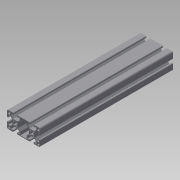
# Autodesk Inventor part: 1530-ULS
Saved by Autodesk Inventor 2013 (Build 170138000, 138)
## iProperties
Created: 2014-04-23
Part Number: 1530-ULS
Material: Generic
Document SubType Name: Modeling
Density: 1 g/cm^3
Vendor: 80/20 Inc.
Engineer: Ross Bowman
Designer: Ross Bowman
Catalog Web Link: 8020.net
Company: 80/20 Inc.
Author: Ross Bowman
Keywords: 80/20 , 8020 , T-Slot , Extrusion
Material: 6105-T5 Aluminum
Autodesk Inventor part; units mm, degrees
ref_plane "YZ Plane" through (0, 0, 0) normal (1, 0, 0) x (0, 1, 0)
ref_plane "XZ Plane" through (0, 0, 0) normal (0, 1, 0) x (-1, 0, 0)
ref_plane "XY Plane" through (0, 0, 0) normal (0, 0, 1) x (1, 0, 0)
sketch "Sketch1" plane through (0, 0, 0) normal (0, 0, 1) x (1, 0, 0)
  arc A0 (30.9118, 12.2428) -> (31.2928, 11.8618) centre (31.2928, 12.2428) ccw
  line L0 (30.9118, 16.8656) -> (30.9118, 12.2428)
  arc A1 (31.2928, 17.2466) -> (30.9118, 16.8656) centre (31.2928, 16.8656) ccw
  line L1 (33.5026, 17.2466) -> (31.2928, 17.2466)
  arc A2 (36.2966, 14.4526) -> (33.5026, 17.2466) centre (33.5026, 14.4526) ccw
  line L2 (36.2966, 12.2428) -> (36.2966, 14.4526)
  arc A3 (35.9156, 11.8618) -> (36.2966, 12.2428) centre (35.9156, 12.2428) ccw
  line L3 (31.2928, 11.8618) -> (35.9156, 11.8618)
  arc A4 (22.1619, -1.178) -> (22.1619, 1.178) centre (19.05, 0) ccw
  arc A5 (22.1619, -1.178) -> (22.2488, -1.5823) centre (22.5182, -1.3129) ccw
  line L4 (23.9585, -3.2921) -> (22.2488, -1.5823)
  arc A6 (24.2189, -3.9207) -> (23.9585, -3.2921) centre (23.3299, -3.9207) ccw
  line L5 (24.2189, -4.9149) -> (24.2189, -3.9207)
  arc A7 (23.9649, -5.1689) -> (24.2189, -4.9149) centre (23.9649, -4.9149) ccw
  line L6 (22.9707, -5.1689) -> (23.9649, -5.1689)
  arc A8 (22.3421, -4.9085) -> (22.9707, -5.1689) centre (22.9707, -4.2799) ccw
  line L7 (20.6323, -3.1988) -> (22.3421, -4.9085)
  arc A9 (20.6323, -3.1988) -> (20.228, -3.1119) centre (20.3629, -3.4682) ccw
  arc A10 (17.872, -3.1119) -> (20.228, -3.1119) centre (19.05, 0) ccw
  arc A11 (17.872, -3.1119) -> (17.4677, -3.1988) centre (17.7371, -3.4682) ccw
  line L8 (15.7579, -4.9085) -> (17.4677, -3.1988)
  arc A12 (15.1293, -5.1689) -> (15.7579, -4.9085) centre (15.1293, -4.2799) ccw
  line L9 (14.1351, -5.1689) -> (15.1293, -5.1689)
  arc A13 (13.8811, -4.9149) -> (14.1351, -5.1689) centre (14.1351, -4.9149) ccw
  line L10 (13.8811, -3.9207) -> (13.8811, -4.9149)
  arc A14 (14.1415, -3.2921) -> (13.8811, -3.9207) centre (14.7701, -3.9207) ccw
  line L11 (15.8512, -1.5823) -> (14.1415, -3.2921)
  arc A15 (15.8512, -1.5823) -> (15.9381, -1.178) centre (15.5818, -1.3129) ccw
  arc A16 (15.9381, 1.178) -> (15.9381, -1.178) centre (19.05, 0) ccw
  arc A17 (15.9381, 1.178) -> (15.8512, 1.5823) centre (15.5818, 1.3129) ccw
  line L12 (14.1415, 3.2921) -> (15.8512, 1.5823)
  arc A18 (13.8811, 3.9207) -> (14.1415, 3.2921) centre (14.7701, 3.9207) ccw
  line L13 (13.8811, 4.9149) -> (13.8811, 3.9207)
  arc A19 (14.1351, 5.1689) -> (13.8811, 4.9149) centre (14.1351, 4.9149) ccw
  line L14 (15.1293, 5.1689) -> (14.1351, 5.1689)
  arc A20 (15.7579, 4.9085) -> (15.1293, 5.1689) centre (15.1293, 4.2799) ccw
  line L15 (17.4677, 3.1988) -> (15.7579, 4.9085)
  arc A21 (17.4677, 3.1988) -> (17.872, 3.1119) centre (17.7371, 3.4682) ccw
  arc A22 (20.228, 3.1119) -> (17.872, 3.1119) centre (19.05, 0) ccw
  arc A23 (20.228, 3.1119) -> (20.6323, 3.1988) centre (20.3629, 3.4682) ccw
  line L16 (22.3421, 4.9085) -> (20.6323, 3.1988)
  arc A24 (22.9707, 5.1689) -> (22.3421, 4.9085) centre (22.9707, 4.2799) ccw
  line L17 (23.9649, 5.1689) -> (22.9707, 5.1689)
  arc A25 (24.2189, 4.9149) -> (23.9649, 5.1689) centre (23.9649, 4.9149) ccw
  line L18 (24.2189, 3.9207) -> (24.2189, 4.9149)
  arc A26 (23.9585, 3.2921) -> (24.2189, 3.9207) centre (23.3299, 3.9207) ccw
  line L19 (22.2488, 1.5823) -> (23.9585, 3.2921)
  arc A27 (22.2488, 1.5823) -> (22.1619, 1.178) centre (22.5182, 1.3129) ccw
  arc A28 (-30.9118, -12.2428) -> (-31.2928, -11.8618) centre (-31.2928, -12.2428) ccw
  line L20 (-30.9118, -16.8656) -> (-30.9118, -12.2428)
  arc A29 (-31.2928, -17.2466) -> (-30.9118, -16.8656) centre (-31.2928, -16.8656) ccw
  line L21 (-33.5026, -17.2466) -> (-31.2928, -17.2466)
  arc A30 (-36.2966, -14.4526) -> (-33.5026, -17.2466) centre (-33.5026, -14.4526) ccw
  line L22 (-36.2966, -12.2428) -> (-36.2966, -14.4526)
  arc A31 (-35.9156, -11.8618) -> (-36.2966, -12.2428) centre (-35.9156, -12.2428) ccw
  line L23 (-31.2928, -11.8618) -> (-35.9156, -11.8618)
  arc A32 (-30.9118, 16.8656) -> (-31.2928, 17.2466) centre (-31.2928, 16.8656) ccw
  line L24 (-30.9118, 12.2428) -> (-30.9118, 16.8656)
  arc A33 (-31.2928, 11.8618) -> (-30.9118, 12.2428) centre (-31.2928, 12.2428) ccw
  line L25 (-35.9156, 11.8618) -> (-31.2928, 11.8618)
  arc A34 (-36.2966, 12.2428) -> (-35.9156, 11.8618) centre (-35.9156, 12.2428) ccw
  line L26 (-36.2966, 14.4526) -> (-36.2966, 12.2428)
  arc A35 (-33.5026, 17.2466) -> (-36.2966, 14.4526) centre (-33.5026, 14.4526) ccw
  line L27 (-31.2928, 17.2466) -> (-33.5026, 17.2466)
  arc A36 (-15.9381, -1.178) -> (-15.9381, 1.178) centre (-19.05, 0) ccw
  arc A37 (-15.9381, -1.178) -> (-15.8512, -1.5823) centre (-15.5818, -1.3129) ccw
  line L28 (-14.1415, -3.2921) -> (-15.8512, -1.5823)
  arc A38 (-13.8811, -3.9207) -> (-14.1415, -3.2921) centre (-14.7701, -3.9207) ccw
  line L29 (-13.8811, -4.9149) -> (-13.8811, -3.9207)
  arc A39 (-14.1351, -5.1689) -> (-13.8811, -4.9149) centre (-14.1351, -4.9149) ccw
  line L30 (-15.1293, -5.1689) -> (-14.1351, -5.1689)
  arc A40 (-15.7579, -4.9085) -> (-15.1293, -5.1689) centre (-15.1293, -4.2799) ccw
  line L31 (-17.4677, -3.1988) -> (-15.7579, -4.9085)
  arc A41 (-17.4677, -3.1988) -> (-17.872, -3.1119) centre (-17.7371, -3.4682) ccw
  arc A42 (-20.228, -3.1119) -> (-17.872, -3.1119) centre (-19.05, 0) ccw
  arc A43 (-20.228, -3.1119) -> (-20.6323, -3.1988) centre (-20.3629, -3.4682) ccw
  line L32 (-22.3421, -4.9085) -> (-20.6323, -3.1988)
  arc A44 (-22.9707, -5.1689) -> (-22.3421, -4.9085) centre (-22.9707, -4.2799) ccw
  line L33 (-23.9649, -5.1689) -> (-22.9707, -5.1689)
  arc A45 (-24.2189, -4.9149) -> (-23.9649, -5.1689) centre (-23.9649, -4.9149) ccw
  line L34 (-24.2189, -3.9207) -> (-24.2189, -4.9149)
  arc A46 (-23.9585, -3.2921) -> (-24.2189, -3.9207) centre (-23.3299, -3.9207) ccw
  line L35 (-22.2488, -1.5823) -> (-23.9585, -3.2921)
  arc A47 (-22.2488, -1.5823) -> (-22.1619, -1.178) centre (-22.5182, -1.3129) ccw
  arc A48 (-22.1619, 1.178) -> (-22.1619, -1.178) centre (-19.05, 0) ccw
  arc A49 (-22.1619, 1.178) -> (-22.2488, 1.5823) centre (-22.5182, 1.3129) ccw
  line L36 (-23.9585, 3.2921) -> (-22.2488, 1.5823)
  arc A50 (-24.2189, 3.9207) -> (-23.9585, 3.2921) centre (-23.3299, 3.9207) ccw
  line L37 (-24.2189, 4.9149) -> (-24.2189, 3.9207)
  arc A51 (-23.9649, 5.1689) -> (-24.2189, 4.9149) centre (-23.9649, 4.9149) ccw
  line L38 (-22.9707, 5.1689) -> (-23.9649, 5.1689)
  arc A52 (-22.3421, 4.9085) -> (-22.9707, 5.1689) centre (-22.9707, 4.2799) ccw
  line L39 (-20.6323, 3.1988) -> (-22.3421, 4.9085)
  arc A53 (-20.6323, 3.1988) -> (-20.228, 3.1119) centre (-20.3629, 3.4682) ccw
  arc A54 (-17.872, 3.1119) -> (-20.228, 3.1119) centre (-19.05, 0) ccw
  arc A55 (-17.872, 3.1119) -> (-17.4677, 3.1988) centre (-17.7371, 3.4682) ccw
  line L40 (-15.7579, 4.9085) -> (-17.4677, 3.1988)
  arc A56 (-15.1293, 5.1689) -> (-15.7579, 4.9085) centre (-15.1293, 4.2799) ccw
  line L41 (-14.1351, 5.1689) -> (-15.1293, 5.1689)
  arc A57 (-13.8811, 4.9149) -> (-14.1351, 5.1689) centre (-14.1351, 4.9149) ccw
  line L42 (-13.8811, 3.9207) -> (-13.8811, 4.9149)
  arc A58 (-14.1415, 3.2921) -> (-13.8811, 3.9207) centre (-14.7701, 3.9207) ccw
  line L43 (-15.8512, 1.5823) -> (-14.1415, 3.2921)
  arc A59 (-15.8512, 1.5823) -> (-15.9381, 1.178) centre (-15.5818, 1.3129) ccw
  arc A60 (6.8072, -17.2466) -> (7.1882, -16.8656) centre (6.8072, -16.8656) ccw
  line L44 (-6.8072, -17.2466) -> (6.8072, -17.2466)
  arc A61 (-7.1882, -16.8656) -> (-6.8072, -17.2466) centre (-6.8072, -16.8656) ccw
  line L45 (-7.1882, -10.8253) -> (-7.1882, -16.8656)
  arc A62 (-7.1882, -10.8253) -> (-7.5602, -9.9273) centre (-8.4582, -10.8253) ccw
  line L46 (-11.9343, -5.5531) -> (-7.5602, -9.9273)
  arc A63 (-12.3063, -4.6551) -> (-11.9343, -5.5531) centre (-11.0363, -4.6551) ccw
  line L47 (-12.3063, 4.6551) -> (-12.3063, -4.6551)
  arc A64 (-11.9343, 5.5531) -> (-12.3063, 4.6551) centre (-11.0363, 4.6551) ccw
  line L48 (-7.5602, 9.9273) -> (-11.9343, 5.5531)
  arc A65 (-7.5602, 9.9273) -> (-7.1882, 10.8253) centre (-8.4582, 10.8253) ccw
  line L49 (-7.1882, 16.8656) -> (-7.1882, 10.8253)
  arc A66 (-6.8072, 17.2466) -> (-7.1882, 16.8656) centre (-6.8072, 16.8656) ccw
  line L50 (6.8072, 17.2466) -> (-6.8072, 17.2466)
  arc A67 (7.1882, 16.8656) -> (6.8072, 17.2466) centre (6.8072, 16.8656) ccw
  line L51 (7.1882, 10.8253) -> (7.1882, 16.8656)
  arc A68 (7.1882, 10.8253) -> (7.5602, 9.9273) centre (8.4582, 10.8253) ccw
  line L52 (11.9343, 5.5531) -> (7.5602, 9.9273)
  arc A69 (12.3063, 4.6551) -> (11.9343, 5.5531) centre (11.0363, 4.6551) ccw
  line L53 (12.3063, -4.6551) -> (12.3063, 4.6551)
  arc A70 (11.9343, -5.5531) -> (12.3063, -4.6551) centre (11.0363, -4.6551) ccw
  line L54 (7.5602, -9.9273) -> (11.9343, -5.5531)
  arc A71 (7.5602, -9.9273) -> (7.1882, -10.8253) centre (8.4582, -10.8253) ccw
  line L55 (7.1882, -16.8656) -> (7.1882, -10.8253)
  arc A72 (30.9118, -16.8656) -> (31.2928, -17.2466) centre (31.2928, -16.8656) ccw
  line L56 (30.9118, -12.2428) -> (30.9118, -16.8656)
  arc A73 (31.2928, -11.8618) -> (30.9118, -12.2428) centre (31.2928, -12.2428) ccw
  line L57 (35.9156, -11.8618) -> (31.2928, -11.8618)
  arc A74 (36.2966, -12.2428) -> (35.9156, -11.8618) centre (35.9156, -12.2428) ccw
  line L58 (36.2966, -14.4526) -> (36.2966, -12.2428)
  arc A75 (33.5026, -17.2466) -> (36.2966, -14.4526) centre (33.5026, -14.4526) ccw
  line L59 (31.2928, -17.2466) -> (33.5026, -17.2466)
  arc A76 (-14.986, -17.4752) -> (-13.4112, -19.05) centre (-13.4112, -17.4752) ccw
  line L60 (-13.4112, -19.05) -> (13.4112, -19.05)
  arc A77 (13.4112, -19.05) -> (14.986, -17.4752) centre (13.4112, -17.4752) ccw
  line L61 (14.986, -17.4752) -> (14.986, -16.5608)
  arc A78 (14.986, -16.5608) -> (13.4112, -14.986) centre (13.4112, -16.5608) ccw
  line L62 (13.4112, -14.986) -> (12.573, -14.986)
  arc A79 (12.573, -14.986) -> (12.192, -15.367) centre (12.573, -15.367) ccw
  line L63 (12.192, -15.367) -> (12.192, -15.6972)
  arc A80 (11.811, -16.0782) -> (12.192, -15.6972) centre (11.811, -15.6972) ccw
  line L64 (11.811, -16.0782) -> (9.652, -16.0782)
  arc A81 (8.763, -15.1892) -> (9.652, -16.0782) centre (9.652, -15.1892) ccw
  line L65 (8.763, -15.1892) -> (8.763, -12.3756)
  arc A82 (9.135, -11.4776) -> (8.763, -12.3756) centre (10.033, -12.3756) ccw
  line L66 (9.135, -11.4776) -> (13.4969, -7.1157)
  arc A83 (14.3949, -6.7437) -> (13.4969, -7.1157) centre (14.3949, -8.0137) ccw
  line L67 (14.3949, -6.7437) -> (23.7051, -6.7437)
  arc A84 (24.6031, -7.1157) -> (23.7051, -6.7437) centre (23.7051, -8.0137) ccw
  line L68 (24.6031, -7.1157) -> (28.965, -11.4776)
  arc A85 (29.337, -12.3756) -> (28.965, -11.4776) centre (28.067, -12.3756) ccw
  line L69 (29.337, -12.3756) -> (29.337, -15.1892)
  arc A86 (28.448, -16.0782) -> (29.337, -15.1892) centre (28.448, -15.1892) ccw
  line L70 (28.448, -16.0782) -> (26.289, -16.0782)
  arc A87 (25.908, -15.6972) -> (26.289, -16.0782) centre (26.289, -15.6972) ccw
  line L71 (25.908, -15.6972) -> (25.908, -15.367)
  arc A88 (25.908, -15.367) -> (25.527, -14.986) centre (25.527, -15.367) ccw
  line L72 (25.527, -14.986) -> (24.6888, -14.986)
  arc A89 (24.6888, -14.986) -> (23.114, -16.5608) centre (24.6888, -16.5608) ccw
  line L73 (23.114, -16.5608) -> (23.114, -17.4752)
  arc A90 (23.114, -17.4752) -> (24.6888, -19.05) centre (24.6888, -17.4752) ccw
  line L74 (24.6888, -19.05) -> (34.925, -19.05)
  arc A91 (34.925, -19.05) -> (38.1, -15.875) centre (34.925, -15.875) ccw
  line L75 (38.1, -15.875) -> (38.1, -5.6388)
  arc A92 (38.1, -5.6388) -> (36.5252, -4.064) centre (36.5252, -5.6388) ccw
  line L76 (36.5252, -4.064) -> (35.6108, -4.064)
  arc A93 (35.6108, -4.064) -> (34.036, -5.6388) centre (35.6108, -5.6388) ccw
  line L77 (34.036, -5.6388) -> (34.036, -6.477)
  arc A94 (34.036, -6.477) -> (34.417, -6.858) centre (34.417, -6.477) ccw
  line L78 (34.417, -6.858) -> (34.7472, -6.858)
  arc A95 (35.1282, -7.239) -> (34.7472, -6.858) centre (34.7472, -7.239) ccw
  line L79 (35.1282, -7.239) -> (35.1282, -9.398)
  arc A96 (34.2392, -10.287) -> (35.1282, -9.398) centre (34.2392, -9.398) ccw
  line L80 (34.2392, -10.287) -> (31.4256, -10.287)
  arc A97 (30.5276, -9.915) -> (31.4256, -10.287) centre (31.4256, -9.017) ccw
  line L81 (30.5276, -9.915) -> (26.1657, -5.5531)
  arc A98 (25.7937, -4.6551) -> (26.1657, -5.5531) centre (27.0637, -4.6551) ccw
  line L82 (25.7937, -4.6551) -> (25.7937, 4.6551)
  arc A99 (26.1657, 5.5531) -> (25.7937, 4.6551) centre (27.0637, 4.6551) ccw
  line L83 (26.1657, 5.5531) -> (30.5276, 9.915)
  arc A100 (31.4256, 10.287) -> (30.5276, 9.915) centre (31.4256, 9.017) ccw
  line L84 (31.4256, 10.287) -> (34.2392, 10.287)
  arc A101 (35.1282, 9.398) -> (34.2392, 10.287) centre (34.2392, 9.398) ccw
  line L85 (35.1282, 9.398) -> (35.1282, 7.239)
  arc A102 (34.7472, 6.858) -> (35.1282, 7.239) centre (34.7472, 7.239) ccw
  line L86 (34.7472, 6.858) -> (34.417, 6.858)
  arc A103 (34.417, 6.858) -> (34.036, 6.477) centre (34.417, 6.477) ccw
  line L87 (34.036, 6.477) -> (34.036, 5.6388)
  arc A104 (34.036, 5.6388) -> (35.6108, 4.064) centre (35.6108, 5.6388) ccw
  line L88 (35.6108, 4.064) -> (36.5252, 4.064)
  arc A105 (36.5252, 4.064) -> (38.1, 5.6388) centre (36.5252, 5.6388) ccw
  line L89 (38.1, 5.6388) -> (38.1, 15.875)
  arc A106 (38.1, 15.875) -> (34.925, 19.05) centre (34.925, 15.875) ccw
  line L90 (34.925, 19.05) -> (24.6888, 19.05)
  arc A107 (24.6888, 19.05) -> (23.114, 17.4752) centre (24.6888, 17.4752) ccw
  line L91 (23.114, 17.4752) -> (23.114, 16.5608)
  arc A108 (23.114, 16.5608) -> (24.6888, 14.986) centre (24.6888, 16.5608) ccw
  line L92 (24.6888, 14.986) -> (25.527, 14.986)
  arc A109 (25.527, 14.986) -> (25.908, 15.367) centre (25.527, 15.367) ccw
  line L93 (25.908, 15.367) -> (25.908, 15.6972)
  arc A110 (26.289, 16.0782) -> (25.908, 15.6972) centre (26.289, 15.6972) ccw
  line L94 (26.289, 16.0782) -> (28.448, 16.0782)
  arc A111 (29.337, 15.1892) -> (28.448, 16.0782) centre (28.448, 15.1892) ccw
  line L95 (29.337, 15.1892) -> (29.337, 12.3756)
  arc A112 (28.965, 11.4776) -> (29.337, 12.3756) centre (28.067, 12.3756) ccw
  line L96 (28.965, 11.4776) -> (24.6031, 7.1157)
  arc A113 (23.7051, 6.7437) -> (24.6031, 7.1157) centre (23.7051, 8.0137) ccw
  line L97 (23.7051, 6.7437) -> (14.3949, 6.7437)
  arc A114 (13.4969, 7.1157) -> (14.3949, 6.7437) centre (14.3949, 8.0137) ccw
  line L98 (13.4969, 7.1157) -> (9.135, 11.4776)
  arc A115 (8.763, 12.3756) -> (9.135, 11.4776) centre (10.033, 12.3756) ccw
  line L99 (8.763, 12.3756) -> (8.763, 15.1892)
  arc A116 (9.652, 16.0782) -> (8.763, 15.1892) centre (9.652, 15.1892) ccw
  line L100 (9.652, 16.0782) -> (11.811, 16.0782)
  arc A117 (12.192, 15.6972) -> (11.811, 16.0782) centre (11.811, 15.6972) ccw
  line L101 (12.192, 15.6972) -> (12.192, 15.367)
  arc A118 (12.192, 15.367) -> (12.573, 14.986) centre (12.573, 15.367) ccw
  line L102 (12.573, 14.986) -> (13.4112, 14.986)
  arc A119 (13.4112, 14.986) -> (14.986, 16.5608) centre (13.4112, 16.5608) ccw
  line L103 (14.986, 16.5608) -> (14.986, 17.4752)
  arc A120 (14.986, 17.4752) -> (13.4112, 19.05) centre (13.4112, 17.4752) ccw
  line L104 (13.4112, 19.05) -> (-13.4112, 19.05)
  arc A121 (-13.4112, 19.05) -> (-14.986, 17.4752) centre (-13.4112, 17.4752) ccw
  line L105 (-14.986, 17.4752) -> (-14.986, 16.5608)
  arc A122 (-14.986, 16.5608) -> (-13.4112, 14.986) centre (-13.4112, 16.5608) ccw
  line L106 (-13.4112, 14.986) -> (-12.573, 14.986)
  arc A123 (-12.573, 14.986) -> (-12.192, 15.367) centre (-12.573, 15.367) ccw
  line L107 (-12.192, 15.367) -> (-12.192, 15.6972)
  arc A124 (-11.811, 16.0782) -> (-12.192, 15.6972) centre (-11.811, 15.6972) ccw
  line L108 (-11.811, 16.0782) -> (-9.652, 16.0782)
  arc A125 (-8.763, 15.1892) -> (-9.652, 16.0782) centre (-9.652, 15.1892) ccw
  line L109 (-8.763, 15.1892) -> (-8.763, 12.3756)
  arc A126 (-9.135, 11.4776) -> (-8.763, 12.3756) centre (-10.033, 12.3756) ccw
  line L110 (-9.135, 11.4776) -> (-13.4969, 7.1157)
  arc A127 (-14.3949, 6.7437) -> (-13.4969, 7.1157) centre (-14.3949, 8.0137) ccw
  line L111 (-14.3949, 6.7437) -> (-23.7051, 6.7437)
  arc A128 (-24.6031, 7.1157) -> (-23.7051, 6.7437) centre (-23.7051, 8.0137) ccw
  line L112 (-24.6031, 7.1157) -> (-28.965, 11.4776)
  arc A129 (-29.337, 12.3756) -> (-28.965, 11.4776) centre (-28.067, 12.3756) ccw
  line L113 (-29.337, 12.3756) -> (-29.337, 15.1892)
  arc A130 (-28.448, 16.0782) -> (-29.337, 15.1892) centre (-28.448, 15.1892) ccw
  line L114 (-28.448, 16.0782) -> (-26.289, 16.0782)
  arc A131 (-25.908, 15.6972) -> (-26.289, 16.0782) centre (-26.289, 15.6972) ccw
  line L115 (-25.908, 15.6972) -> (-25.908, 15.367)
  arc A132 (-25.908, 15.367) -> (-25.527, 14.986) centre (-25.527, 15.367) ccw
  line L116 (-25.527, 14.986) -> (-24.6888, 14.986)
  arc A133 (-24.6888, 14.986) -> (-23.114, 16.5608) centre (-24.6888, 16.5608) ccw
  line L117 (-23.114, 16.5608) -> (-23.114, 17.4752)
  arc A134 (-23.114, 17.4752) -> (-24.6888, 19.05) centre (-24.6888, 17.4752) ccw
  line L118 (-24.6888, 19.05) -> (-34.925, 19.05)
  arc A135 (-34.925, 19.05) -> (-38.1, 15.875) centre (-34.925, 15.875) ccw
  line L119 (-38.1, 15.875) -> (-38.1, 5.6388)
  arc A136 (-38.1, 5.6388) -> (-36.5252, 4.064) centre (-36.5252, 5.6388) ccw
  line L120 (-36.5252, 4.064) -> (-35.6108, 4.064)
  arc A137 (-35.6108, 4.064) -> (-34.036, 5.6388) centre (-35.6108, 5.6388) ccw
  line L121 (-34.036, 5.6388) -> (-34.036, 6.477)
  arc A138 (-34.036, 6.477) -> (-34.417, 6.858) centre (-34.417, 6.477) ccw
  line L122 (-34.417, 6.858) -> (-34.7472, 6.858)
  arc A139 (-35.1282, 7.239) -> (-34.7472, 6.858) centre (-34.7472, 7.239) ccw
  line L123 (-35.1282, 7.239) -> (-35.1282, 9.398)
  arc A140 (-34.2392, 10.287) -> (-35.1282, 9.398) centre (-34.2392, 9.398) ccw
  line L124 (-34.2392, 10.287) -> (-31.4256, 10.287)
  arc A141 (-30.5276, 9.915) -> (-31.4256, 10.287) centre (-31.4256, 9.017) ccw
  line L125 (-30.5276, 9.915) -> (-26.1657, 5.5531)
  arc A142 (-25.7937, 4.6551) -> (-26.1657, 5.5531) centre (-27.0637, 4.6551) ccw
  line L126 (-25.7937, 4.6551) -> (-25.7937, -4.6551)
  arc A143 (-26.1657, -5.5531) -> (-25.7937, -4.6551) centre (-27.0637, -4.6551) ccw
  line L127 (-26.1657, -5.5531) -> (-30.5276, -9.915)
  arc A144 (-31.4256, -10.287) -> (-30.5276, -9.915) centre (-31.4256, -9.017) ccw
  line L128 (-31.4256, -10.287) -> (-34.2392, -10.287)
  arc A145 (-35.1282, -9.398) -> (-34.2392, -10.287) centre (-34.2392, -9.398) ccw
  line L129 (-35.1282, -9.398) -> (-35.1282, -7.239)
  arc A146 (-34.7472, -6.858) -> (-35.1282, -7.239) centre (-34.7472, -7.239) ccw
  line L130 (-34.7472, -6.858) -> (-34.417, -6.858)
  arc A147 (-34.417, -6.858) -> (-34.036, -6.477) centre (-34.417, -6.477) ccw
  line L131 (-34.036, -6.477) -> (-34.036, -5.6388)
  arc A148 (-34.036, -5.6388) -> (-35.6108, -4.064) centre (-35.6108, -5.6388) ccw
  line L132 (-35.6108, -4.064) -> (-36.5252, -4.064)
  arc A149 (-36.5252, -4.064) -> (-38.1, -5.6388) centre (-36.5252, -5.6388) ccw
  line L133 (-38.1, -5.6388) -> (-38.1, -15.875)
  arc A150 (-38.1, -15.875) -> (-34.925, -19.05) centre (-34.925, -15.875) ccw
  line L134 (-34.925, -19.05) -> (-24.6888, -19.05)
  arc A151 (-24.6888, -19.05) -> (-23.114, -17.4752) centre (-24.6888, -17.4752) ccw
  line L135 (-23.114, -17.4752) -> (-23.114, -16.5608)
  arc A152 (-23.114, -16.5608) -> (-24.6888, -14.986) centre (-24.6888, -16.5608) ccw
  line L136 (-24.6888, -14.986) -> (-25.527, -14.986)
  arc A153 (-25.527, -14.986) -> (-25.908, -15.367) centre (-25.527, -15.367) ccw
  line L137 (-25.908, -15.367) -> (-25.908, -15.6972)
  arc A154 (-26.289, -16.0782) -> (-25.908, -15.6972) centre (-26.289, -15.6972) ccw
  line L138 (-26.289, -16.0782) -> (-28.448, -16.0782)
  arc A155 (-29.337, -15.1892) -> (-28.448, -16.0782) centre (-28.448, -15.1892) ccw
  line L139 (-29.337, -15.1892) -> (-29.337, -12.3756)
  arc A156 (-28.965, -11.4776) -> (-29.337, -12.3756) centre (-28.067, -12.3756) ccw
  line L140 (-28.965, -11.4776) -> (-24.6031, -7.1157)
  arc A157 (-23.7051, -6.7437) -> (-24.6031, -7.1157) centre (-23.7051, -8.0137) ccw
  line L141 (-23.7051, -6.7437) -> (-14.3949, -6.7437)
  arc A158 (-13.4969, -7.1157) -> (-14.3949, -6.7437) centre (-14.3949, -8.0137) ccw
  line L142 (-13.4969, -7.1157) -> (-9.135, -11.4776)
  arc A159 (-8.763, -12.3756) -> (-9.135, -11.4776) centre (-10.033, -12.3756) ccw
  line L143 (-8.763, -12.3756) -> (-8.763, -15.1892)
  arc A160 (-9.652, -16.0782) -> (-8.763, -15.1892) centre (-9.652, -15.1892) ccw
  line L144 (-9.652, -16.0782) -> (-11.811, -16.0782)
  arc A161 (-12.192, -15.6972) -> (-11.811, -16.0782) centre (-11.811, -15.6972) ccw
  line L145 (-12.192, -15.6972) -> (-12.192, -15.367)
  arc A162 (-12.192, -15.367) -> (-12.573, -14.986) centre (-12.573, -15.367) ccw
  line L146 (-12.573, -14.986) -> (-13.4112, -14.986)
  arc A163 (-13.4112, -14.986) -> (-14.986, -16.5608) centre (-13.4112, -16.5608) ccw
  line L147 (-14.986, -16.5608) -> (-14.986, -17.4752)
  point P0 (0, 0)
  constraints: 328 point on circle, 296 end point, 164 centre point
extrude "Extrusion1" add sketch "Sketch1" against normal blind 304.8
body "Solid1"
